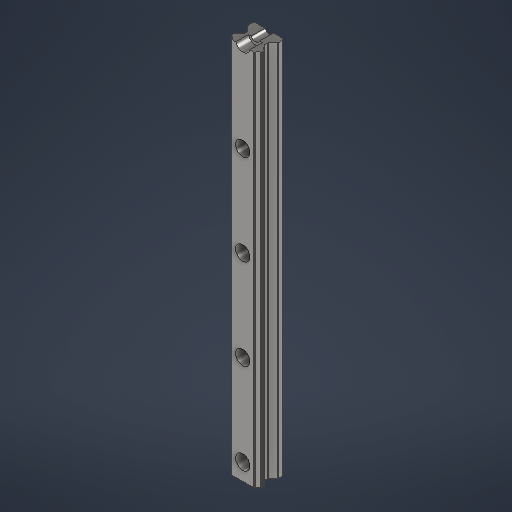
# Autodesk Inventor part: HGR20R-LinearRail200mm
Saved by Autodesk Inventor 2026.2 (Build 302298000, 298)
## iProperties
Created: 2026-06-19
Part Number: HGR20R-LinearRail200mm
Material: Stainless Steel
Document SubType Name: Modeling
Designer: Kenji
Density: 8 g/cm^3
Appearance: Semi-Polished
Author: Kenji
Autodesk Inventor part; units mm, degrees
ref_plane "YZ Plane" through (0, 0, 0) normal (1, 0, 0) x (0, 1, 0)
ref_plane "XZ Plane" through (0, 0, 0) normal (0, 1, 0) x (-1, 0, 0)
ref_plane "XY Plane" through (0, 0, 0) normal (0, 0, 1) x (1, 0, 0)
sketch "Sketch1" plane through (0, 0, 0) normal (0, 1, 0) x (-1, 0, 0)
  arc A0 (-6.7759, -1.5867) -> (-6.483, -0.8796) centre (-7.483, -0.8796) ccw
  line L0 (-7.1187, 8.7305) -> (7.3527, 8.7305)
  line L1 (9.117, -8.7695) -> (-8.883, -8.7695)
  line L2 (6.717, 0.6806) -> (6.717, -0.8796)
  arc A1 (7.0099, 1.3877) -> (6.717, 0.6806) centre (7.717, 0.6806) ccw
  line L3 (7.7471, 2.1249) -> (7.0099, 1.3877)
  arc A2 (6.717, -0.8796) -> (7.0099, -1.5867) centre (7.717, -0.8796) ccw
  arc A3 (-9.5901, -4.4009) -> (-9.883, -5.108) centre (-8.883, -5.108) ccw
  line L4 (-9.883, -7.7695) -> (-9.883, -5.108)
  line L5 (-8.883, -8.7695) -> (-9.883, -7.7695)
  line L6 (-9.5901, -4.4009) -> (-6.7759, -1.5867)
  line L7 (10.117, 5.7591) -> (10.117, 4.7019)
  arc A4 (10.117, 5.7591) -> (9.9705, 6.1127) centre (9.617, 5.7591) ccw
  line L8 (9.8076, 6.2756) -> (9.9705, 6.1127)
  arc A5 (9.8076, 6.2756) -> (9.5394, 6.4246) centre (9.4424, 5.9341) ccw
  arc A6 (7.9651, 7.9985) -> (9.5394, 6.4246) centre (9.9271, 8.3866) ccw
  arc A7 (7.9651, 7.9985) -> (7.7495, 8.3337) centre (7.4717, 7.918) ccw
  line L9 (7.3527, 8.7305) -> (7.7495, 8.3337)
  line L10 (-6.483, -0.8796) -> (-6.483, 0.6806)
  arc A8 (-6.483, 0.6806) -> (-6.7759, 1.3877) centre (-7.483, 0.6806) ccw
  line L11 (-6.7759, 1.3877) -> (-7.5132, 2.1249)
  arc A9 (-7.7298, 2.463) -> (-7.5132, 2.1249) centre (-7.2359, 2.541) ccw
  arc A10 (-7.7298, 2.463) -> (-9.3148, 4.048) centre (-9.6936, 2.0842) ccw
  line L12 (-9.5736, 4.1854) -> (-9.7366, 4.3483)
  arc A11 (-9.883, 4.7019) -> (-9.7366, 4.3483) centre (-9.383, 4.7019) ccw
  line L13 (-9.883, 4.7019) -> (-9.883, 5.7591)
  arc A12 (-9.7366, 6.1127) -> (-9.883, 5.7591) centre (-9.383, 5.7591) ccw
  arc A13 (9.9705, 4.3483) -> (10.117, 4.7019) centre (9.617, 4.7019) ccw
  line L14 (9.9705, 4.3483) -> (9.8076, 4.1854)
  arc A14 (9.5488, 4.048) -> (9.8076, 4.1854) centre (9.4541, 4.539) ccw
  arc A15 (9.5488, 4.048) -> (7.9638, 2.463) centre (9.9276, 2.0842) ccw
  arc A16 (7.7471, 2.1249) -> (7.9638, 2.463) centre (7.4699, 2.541) ccw
  line L15 (7.0099, -1.5867) -> (9.8241, -4.4009)
  arc A17 (10.117, -5.108) -> (9.8241, -4.4009) centre (9.117, -5.108) ccw
  line L16 (10.117, -5.108) -> (10.117, -7.7695)
  line L17 (10.117, -7.7695) -> (9.117, -8.7695)
  line L18 (-9.7366, 6.1127) -> (-9.5736, 6.2756)
  arc A18 (-9.3054, 6.4246) -> (-9.5736, 6.2756) centre (-9.2085, 5.9341) ccw
  arc A19 (-9.3054, 6.4246) -> (-7.7312, 7.9985) centre (-9.6932, 8.3866) ccw
  arc A20 (-7.5156, 8.3337) -> (-7.7312, 7.9985) centre (-7.2377, 7.918) ccw
  line L19 (-7.5156, 8.3337) -> (-7.1187, 8.7305)
  arc A21 (-9.5736, 4.1854) -> (-9.3148, 4.048) centre (-9.2201, 4.539) ccw
  point P0 (0, 0)
  point P1 (0.117, -0.039)
  point P2 (0.117, 5.2305)
  constraints: 44 point on circle, 40 end point, 22 centre point, 6 vertical, 2 horizontal, 100 other
extrude "Extrusion1" add sketch "Sketch1" along normal blind 250
sketch "Sketch2" plane through (-7.3527, 0, 8.7305) normal (0, 0, 1) x (1, 0, 0)
  circle A0 centre (7.2357, 11.1125) radius 3
  line L0 (0, 0) -> (14.4714, 0) projected
  line L1 (-2.7643, 0) -> (-2.7643, 250) projected
  line L2 (17.2357, 0) -> (17.2357, 250) projected
  circle A1 centre (7.2357, 71.1125) radius 3
  circle A2 centre (7.2357, 131.1125) radius 3
  circle A3 centre (7.2357, 191.1125) radius 3
  circle A4 centre (7.2357, 251.1125) radius 3
  point P0 (7.3527, 0)
  dimension "d2" = 6
  dimension "d3" = 11.1125
  dimension "d4" = 20
  dimension "d5" = 10
  dimension "d8" = 60
  dimension "d18" = 60
  constraints: 5 centre point, 1 equal radius, 1 vertical, 1 vertical alignment, 6 other
  measures "d2" diameter of A0
  measures "d3" distance from line of L0 A0.centre
  measures "d4" distance between parallel lines of L1 L2
  measures "d5" distance from line of A0.centre L2
  measures "d8" distance of A0.centre A1.centre
  measures "d18" distance of A4.centre A3.centre
extrude "Extrusion2" cut sketch "Sketch2" against normal through all contours A0 | A1 | A2 | A3
sketch "Sketch3" plane through (-7.3527, 0, 8.7305) normal (0, 0, 1) x (1, 0, 0)
  circle A0 centre (7.2357, 71.1125) radius 3 projected
  circle A1 centre (7.2357, 131.1125) radius 3 projected
  circle A2 centre (7.2357, 11.1125) radius 3 projected
  circle A3 centre (7.2357, 191.1125) radius 3 projected
  line L0 (0, 0) -> (14.4714, 0) projected
  line L1 (14.4714, 0) -> (14.4714, 250) projected
  line L2 (0, 250) -> (14.4714, 250) projected
  line L3 (0, 0) -> (0, 250) projected
  circle A4 centre (7.2357, 11.1125) radius 4.75
  circle A5 centre (7.2357, 71.1125) radius 4.75
  circle A6 centre (7.2357, 131.1125) radius 4.75
  circle A7 centre (7.2357, 191.1125) radius 4.75
  circle A8 centre (7.2357, 251.1125) radius 4.75
  point P0 (7.3527, 0)
  point P1 (11.8536, 250)
  point P2 (2.6178, 250)
  dimension "d15" = 9.5
  dimension "d21" = 60
  constraints: 5 centre point, 4 coincident, 4 equal radius, 1 vertical alignment
  measures "d15" diameter of A4
  measures "d21" distance of A8.centre A3.centre
extrude "Extrusion3" cut sketch "Sketch3" against normal blind 8.4 contours A4 | A5 | A6 | A7
extrude "Extrusion4" cut sketch "Sketch2" against normal through all contours A4
extrude "Extrusion5" cut sketch "Sketch3" against normal up to surface (8.4 mm away) contours L2 A8 picked at (8.3547, 248.0358)
equation "\"d5\" = 0.5 * d4"
body "Solid1"
